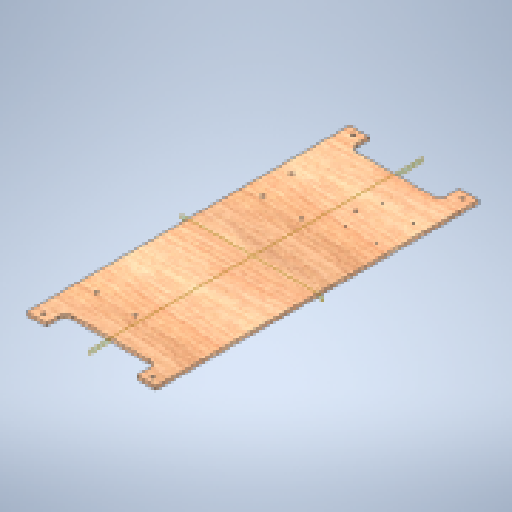
# Autodesk Inventor part: Base_Plate
Saved by Autodesk Inventor 2025.1 (Build 291241020, 241B)
## iProperties
Created: 2024-11-13
Part Number: Base_Plate
Material: Wood (Birch)
Document SubType Name: Modeling
Designer: leon-
Density: 0.55 g/cm^3
Appearance: Birch - Natural Polished
Mass: 251.666 g
Surface Area: 1913.04 cm^2
Volume: 457.575 cm^3
Author: leon-
Autodesk Inventor part; units mm, degrees
ref_plane "YZ Plane" through (0, 0, 0) normal (1, 0, 0) x (0, 1, 0)
ref_plane "XZ Plane" through (0, 0, 0) normal (0, 1, 0) x (-1, 0, 0)
ref_plane "XY Plane" through (0, 0, 0) normal (0, 0, 1) x (1, 0, 0)
sketch "Sketch1" plane through (0, 0, 0) normal (0, 1, 0) x (-1, 0, 0)
  line L0 (0, 0) -> (200, 0)
  line L1 (200, 0) -> (200, 440)
  line L2 (200, 440) -> (0, 440)
  line L3 (0, 440) -> (0, 0)
  dimension "d0" = 440
  dimension "d1" = 200
  constraints: 8 end point, 2 parallel, 1 horizontal, 1 perpendicular
  measures "d0" distance of L2.end L0.start
  measures "d1" distance between parallel lines of L1 L3
extrude "Extrusion1" add sketch "Sketch1" along normal blind 5
sketch "Sketch2" plane through (0, 5, 0) normal (0, 1, 0) x (1, 0, 0)
  line L0 (0, -440) -> (0, 0) projected
  line L1 (0, 0) -> (-30, 0)
  line L2 (-30, 0) -> (-30, 30)
  line L3 (-30, 30) -> (0, 30)
  line L4 (0, 30) -> (0, 0)
  point P0 (-30, 15)
  dimension "d4" = 30
  dimension "d5" = 30
  constraints: 8 end point, 2 parallel, 1 horizontal, 1 midpoint, 1 perpendicular
  measures "d4" distance from line of point (-30, 15) L4
  measures "d5" distance between parallel lines of L1 L3
extrude "Extrusion2" add sketch "Sketch2" against normal up to surface (5 mm away)
sketch "Sketch3" plane through (0, 5, 0) normal (0, 1, 0) x (1, 0, 0)
  line L0 (0, 30) -> (-30, 30) projected
  line L1 (0, -440) -> (0, 30) projected
  point P0 (0, 0)
  point P1 (-15, 20)
  dimension "d8" = 10
  dimension "d9" = 15
  measures "d8" distance from line of L0 point (-15, 20)
  measures "d9" distance from line of L1 point (-15, 20)
hole "Hole1" at (-15, 5, -20) direction (0, -1, 0) diameter 5 end through all
ref_plane "Work Plane1" through (-100, 0, 0) normal (-1, 0, 0) x (0, 0, 1)
ref_plane "Work Plane2" through (-200, 0, 220) normal (0, 0, -1) x (-1, 0, 0)
mirror "Mirror1" about plane through (-100, 0, 0) normal (-1, 0, 0) of "Hole1", "Extrusion2"
mirror "Mirror2" about plane through (-200, 0, 220) normal (0, 0, -1) of "Hole1", "Extrusion2", "Mirror1"
fillet "Fillet1" radius 10 4 edges at (-30, 2.5, 0) (-170, 2.5, 0) (-170, 2.5, 440) (-30, 2.5, 440)
sketch "Sketch4" plane through (0, 5, 0) normal (0, 1, 0) x (1, 0, 0)
  line L0 (-200, -470) -> (-200, 30) projected
  line L1 (-40, 0) -> (-160, 0) projected
  point P0 (0, 0)
  point P1 (-112.5, -132.075)
  dimension "d18" = 87.5
  dimension "d19" = 132.075
  measures "d18" distance from line of L0 point (-112.5, -132.075)
  measures "d19" distance from line of L1 point (-112.5, -132.075)
hole "Hole2" at (-112.5, 5, 132.075) direction (0, -1, 0) diameter 5 depth 8 tip angle 118
pattern_linear "Rectangular Pattern1" count 2 spacing 258.115 along (0, 0, 1) count 2 spacing 60 along (-1, 0, 0) of "Hole2"
sketch "Sketch6" plane through (0, 5, 0) normal (0, 1, 0) x (1, 0, 0)
  line L0 (-40, 0) -> (-160, 0) projected
  line L1 (0, 30) -> (0, -470) projected
  point P0 (0, 0)
  point P1 (-20, -50)
  point P2 (-69, -50)
  point P3 (-69, -108)
  point P4 (-20, -108)
  dimension "d35" = 58
  dimension "d36" = 49
  dimension "d37" = 50
  dimension "d38" = 20
  constraints: 2 horizontal alignment, 2 vertical alignment
  measures "d35" distance of point (-20, -50) point (-20, -108)
  measures "d36" distance of point (-69, -50) point (-20, -50)
  measures "d37" distance from line of L0 point (-20, -50)
  measures "d38" distance from line of L1 point (-20, -50)
hole "Hole3" at (-20, 5, 50) at (-69, 5, 50) at (-69, 5, 108) at (-20, 5, 108) direction (0, -1, 0) diameter 2.1 end through all
sketch "Sketch7" plane through (0, 5, 0) normal (0, 1, 0) x (1, 0, 0)
  line L0 (-40, 0) -> (-160, 0) projected
  line L1 (-200, -470) -> (-200, 30) projected
  line L2 (-160, -440) -> (-40, -440) projected
  point P0 (0, 0)
  point P1 (-70, -420)
  point P2 (-170, -420)
  dimension "d46" = 100
  dimension "d56" = 20
  dimension "d57" = 30
  constraints: 1 horizontal alignment
  measures "d46" distance of point (-170, -420) point (-70, -420)
  measures "d56" distance from line of L2 point (-170, -420)
  measures "d57" distance from line of L1 point (-170, -420)
hole "Hole4" at (-70, 5, 420) at (-170, 5, 420) direction (0, -1, 0) diameter 5 end through all
body "Solid1"
